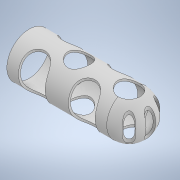
# Autodesk Inventor part: Finger
Saved by Autodesk Inventor 2020 (Build 240168000, 168)
## iProperties
Created: 2020-06-14
Part Number: Finger
Material: Generic
Document SubType Name: Modeling
Designer: maple
Density: 1 g/cm^3
Appearance: Default
Author: maple
Autodesk Inventor part; units mm, degrees
ref_plane "YZ Plane" through (0, 0, 0) normal (1, 0, 0) x (0, 1, 0)
ref_plane "XZ Plane" through (0, 0, 0) normal (0, 1, 0) x (-1, 0, 0)
ref_plane "XY Plane" through (0, 0, 0) normal (0, 0, 1) x (1, 0, 0)
sketch "Sketch1" plane through (0, 0, 0) normal (0, 1, 0) x (-1, 0, 0)
  circle A0 centre (0, 0) radius 11.5
  line L0 (-11.5, 0) -> (51.5, 0)
  line L1 (0, -11.5) -> (51.5, -11.5)
  line L2 (51.5, -11.5) -> (51.5, 0)
  line L3 (0, -11.5) -> (0, -10.5)
  circle A1 centre (0, 0) radius 10.5
  line L4 (0, -10.5) -> (51.5, -10.5)
  line L5 (51.5, -11.5) -> (51.5, -10.5)
  point P0 (-10.5, 0)
  dimension "d0" = 23
  dimension "d1" = 63
  dimension "d2" = 1
  constraints: 12 end point, 3 horizontal, 2 coincident, 2 perpendicular, 2 point on circle, 1 centre point, 1 collinear, 1 point on line, 1 tangent, 1 vertical, 3 other
  measures "d0" diameter of A0
  measures "d1" distance of L0.start L0.end
  measures "d2" distance of L1.start L3.end
revolve "Revolution1" add sketch "Sketch1" angle 360 about axis through (11.5, 0, 0) along (-1, 0, 0) contours L0 A1 L3 A0 | L4 L2 L1 A0 | A0 L3 L4
sketch "Sketch2" plane through (0, 0, 0) normal (0, 1, 0) x (-1, 0, 0)
  line L0 (0, 11.5) -> (0, -11.5) projected
  line L1 (51.5, 11.5) -> (51.5, -11.5) projected
  line L2 (0, 11.5) -> (51.5, 11.5)
  line L3 (0, -11.5) -> (51.5, -11.5)
  line L4 (51.5, 11.5) -> (0, 11.5) projected
  line L5 (25.75, 11.5) -> (0, 11.5)
  line L6 (25.75, 11.5) -> (12.875, 11.5)
  line L7 (25.75, 11.5) -> (51.5, 11.5)
  line L8 (25.75, 11.5) -> (38.625, 11.5)
  line L9 (0, 11.5) -> (6, 11.5)
  circle A0 centre (12.875, 11.5) radius 6.875
  line L10 (51.5, 11.5) -> (45.5, 11.5)
  circle A1 centre (38.625, 11.5) radius 6.875
  line L11 (0, -11.5) -> (25.75, -11.5)
  line L12 (51.5, -11.5) -> (0, -11.5) projected
  line L13 (25.75, -11.5) -> (12.875, -11.5)
  line L14 (25.75, -11.5) -> (51.5, -11.5)
  line L15 (51.5, -11.5) -> (38.625, -11.5)
  line L16 (51.5, -11.5) -> (45.5, -11.5)
  line L17 (0, -11.5) -> (6, -11.5)
  circle A2 centre (12.875, -11.5) radius 6.875
  circle A3 centre (38.625, -11.5) radius 6.875
  line L18 (0, 0) -> (-8.1317, -8.1317)
  arc A4 (0, 11.5) -> (0, -11.5) centre (0, 0) ccw projected
  line L19 (0, 0) -> (11.5, 0) construction
  line L20 (0, 0) -> (-8.1317, 8.1317)
  line L21 (0, 0) -> (11.5, 0) construction
  circle A5 centre (-8.1317, -8.1317) radius 2.5
  circle A6 centre (-8.1317, 8.1317) radius 2.5
  circle A7 centre (-11.5, 0) radius 2.5
  circle A8 centre (0, 0) radius 5.75
  circle A9 centre (25.75, 0) radius 5.75
  dimension "d4" = 6
  dimension "d5" = 6
  dimension "d6" = 6
  dimension "d7" = 6
  dimension "d8" = 135
  dimension "d9" = 135
  dimension "d10" = 5
  dimension "d11" = 5
  dimension "d12" = 5
  constraints: 36 end point, 7 coincident, 6 midpoint, 5 centre point, 4 horizontal, 4 horizontal alignment, 4 point on line, 2 collinear, 2 equal length, 12 other
  measures "d4" distance of L4.end L9.end
  measures "d5" distance of L4.start L10.end
  measures "d6" distance of L12.start L16.end
  measures "d7" distance of L12.end L17.end
  measures "d8" angle of L18 L19
  measures "d9" angle of L21 L20
  measures "d10" diameter of A5
  measures "d11" diameter of A6
  measures "d12" diameter of A7
extrude "Extrusion1" cut sketch "Sketch2" along normal mid plane 63 contours A8 L0 | L0 L20 A8 | A0 L2 | L2 A0 | A6 L20 A4 | A4 A6 | L0 A8 L18 | L18 A8 L20 | L20 A6 A4 | A7 A4 | A4 A7 | A5 A4 L18 | L18 A4 A5 | A1 L2 | L2 A1 | A2 L3 | L3 A2 | A5 A4 | A3 L3 | L3 A3 | A9
body "Solid1"
